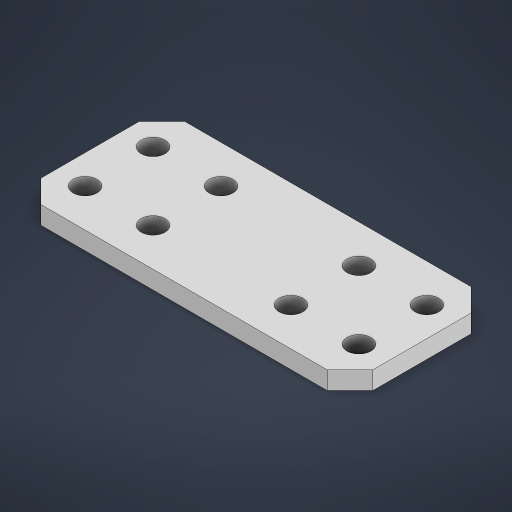
# Autodesk Inventor part: MotorMoutningTopConnectionPlate
Saved by Autodesk Inventor 2024 (Build 280153000, 153)
## iProperties
Created: 2024-01-06
Part Number: MotorMoutningTopConnectionPlate
Material: Generic
Document SubType Name: Modeling
Designer: avsar
Density: 1 g/cm^3
Appearance: Default
Author: avsar
Autodesk Inventor part; units mm, degrees
ref_plane "YZ Plane" through (0, 0, 0) normal (1, 0, 0) x (0, 1, 0)
ref_plane "XZ Plane" through (0, 0, 0) normal (0, 1, 0) x (-1, 0, 0)
ref_plane "XY Plane" through (0, 0, 0) normal (0, 0, 1) x (1, 0, 0)
sketch "Sketch1" plane through (0, 0, 0) normal (0, 1, 0) x (-1, 0, 0)
  circle A0 centre (18.175, 0) radius 2.5 construction
  circle A1 centre (-18.175, 0) radius 2.5 construction
  line L0 (18.175, 0) -> (-18.175, 0) construction
  circle A2 centre (12.175, 6) radius 2.1
  circle A3 centre (12.175, -6) radius 2.1
  circle A4 centre (24.175, -6) radius 2.1
  circle A5 centre (24.175, 6) radius 2.1
  circle A6 centre (-24.175, -6) radius 2.1
  circle A7 centre (-12.175, -6) radius 2.1
  circle A8 centre (-12.175, 6) radius 2.1
  circle A9 centre (-24.175, 6) radius 2.1
  line L1 (29.3, 12.7) -> (-29.3, 12.7)
  line L2 (-29.3, 12.7) -> (-29.3, -12.7)
  line L3 (-29.3, -12.7) -> (29.3, -12.7)
  line L4 (29.3, -12.7) -> (29.3, 12.7)
  line L5 (29.3, 12.7) -> (-29.3, -12.7) construction
  line L6 (-29.3, 12.7) -> (29.3, -12.7) construction
  point P0 (0, 0)
  point P1 (0, 0)
  dimension "d0" = 5
  dimension "d1" = 5
  dimension "d2" = 36.35
  dimension "d3" = 4.2
  dimension "d4" = 6
  dimension "d5" = 6
  dimension "d8" = 360
  dimension "d10" = 4.2
  dimension "d11" = 6
  dimension "d12" = 6
  dimension "d15" = 360
  dimension "d17" = 58.6
  dimension "d18" = 25.4
  constraints: 14 end point, 10 centre point, 3 midpoint, 2 horizontal, 2 parallel, 1 coincident, 1 perpendicular, 18 other
  measures "d0" diameter of A0
  measures "d1" diameter of A1
  measures "d2" distance of L0.start L0.end
  measures "d3" diameter of A2
  measures "d4" horizontal distance of L0.start A2.centre
  measures "d5" horizontal distance of A2.centre L0.start
  measures "d10" diameter of A6
  measures "d11" horizontal distance of A6.centre L0.end
  measures "d12" horizontal distance of L0.end A6.centre
  measures "d17" distance of L3.end L2.end
  measures "d18" distance of L2.end L1.end
extrude "Extrusion1" add sketch "Sketch1" along normal blind 3.175
chamfer "Chamfer1" distance 4 angle 45 4 edges at (-29.3, 1.5875, 12.7) (29.3, 1.5875, 12.7) (29.3, 1.5875, -12.7) (-29.3, 1.5875, -12.7)
body "Solid1"
